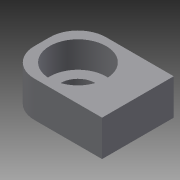
# Autodesk Inventor part: acmeBearingBlock
Saved by Autodesk Inventor 2013 (Build 170138000, 138)
## iProperties
Created: 2012-12-06
Part Number: acmeBearingBlock
Material: Generic
Document SubType Name: Modeling
Designer: Istvan
Density: 1 g/cm^3
Mass: 25.6178 g
Surface Area: 70.9423 cm^2
Volume: 25.6178 cm^3
Author: Istvan
Autodesk Inventor part; units mm, degrees
ref_plane "YZ Plane" through (0, 0, 0) normal (1, 0, 0) x (0, 1, 0)
ref_plane "XZ Plane" through (0, 0, 0) normal (0, 1, 0) x (-1, 0, 0)
ref_plane "XY Plane" through (0, 0, 0) normal (0, 0, 1) x (1, 0, 0)
sketch "Sketch1" plane through (0, 0, 0) normal (0, 1, 0) x (-1, 0, 0)
  line L0 (0, 0) -> (50.927, 0)
  line L1 (50.927, 0) -> (50.927, 38.1)
  line L2 (50.927, 38.1) -> (0, 38.1)
  line L3 (0, 38.1) -> (0, 0)
  dimension "d0" = 50.927
  dimension "d1" = 38.1
  constraints: 8 end point, 2 parallel, 1 horizontal, 1 perpendicular
  measures "d0" distance of L2.end L1.end
  measures "d1" distance of L1.end L0.end
extrude "Extrusion1" add sketch "Sketch1" along normal blind 19.05
sketch "Sketch2" plane through (0, 19.05, 0) normal (0, 1, 0) x (1, 0, 0)
  circle A0 centre (-31.877, -19.05) radius 15
  line L0 (-50.927, -38.1) -> (0, -38.1) projected
  point P0 (-50.927, 0)
  dimension "d4" = 30
  dimension "d5" = 19.05
  dimension "d6" = 19.05
  dimension "d15" = 19.05
  constraints: 1 centre point
  measures "d4" diameter of A0
  measures "d5" horizontal distance of point (-50.927, 0) A0.centre
  measures "d6" horizontal distance of point (-50.927, 0) A0.centre
  measures "d15" distance from line of L0 A0.centre
extrude "Extrusion2" cut sketch "Sketch2" against normal blind 14
sketch "Sketch3" plane through (-31.877, 5.05, 19.05) normal (0, 1, 0) x (1, 0, 0)
  circle A0 centre (0, 0) radius 15 projected
  circle A1 centre (0, 0) radius 3.175
  circle A2 centre (0, 0) radius 9.0875
  point P0 (31.877, 19.05)
  dimension "d9" = 6.35
  dimension "d12" = 5.9125
  dimension "d13" = 5.9125
  constraints: 2 centre point, 2 coincident
  measures "d9" diameter of A1
  measures "d12" radial gap between concentric circles of A2 A1
  measures "d13" radial gap between concentric circles of A0 A2
extrude "Extrusion3" cut sketch "Sketch3" against normal through all contours A1 | A2
fillet "Fillet1" radius 15 2 edges at (-50.927, 9.525, 0) (-50.927, 9.525, 38.1)
equation "\"d5\" = d15"
equation "\"d6\" = d15"
equation "\"d12\" = d13"
body "Solid1"
